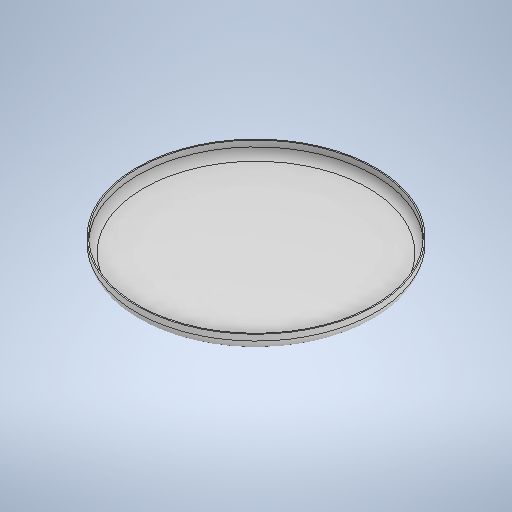
# Autodesk Inventor part: Сферическое дно D1000
Saved by Autodesk Inventor 2025 (Build 290162010, 162A)
## iProperties
Created: 2025-02-16
Part Number: Сферическое дно D1000
Material: Generic
Document SubType Name: Modeling
Designer: pokla
Density: 1 g/cm^3
Appearance: Default
Author: pokla
Autodesk Inventor part; units mm, degrees
ref_plane "YZ Plane" through (0, 0, 0) normal (1, 0, 0) x (0, 1, 0)
ref_plane "XZ Plane" through (0, 0, 0) normal (0, 1, 0) x (-1, 0, 0)
ref_plane "XY Plane" through (0, 0, 0) normal (0, 0, 1) x (1, 0, 0)
sketch "Sketch1" plane through (0, 0, 0) normal (0, 1, 0) x (-1, 0, 0)
  line L0 (606, 0) -> (606, -30)
  arc A0 (571.724, -77.4632) -> (606, -30) centre (556, -30) ccw
  arc A1 (0, -169.7009) -> (571.724, -77.4632) centre (0, 1648.2991) ccw
  line L1 (0, 191.6842) -> (0, -191.6842)
  arc A2 (0, -163.7009) -> (569.8371, -71.7676) centre (0, 1648.2991) ccw
  arc A3 (569.8371, -71.7676) -> (600, -30) centre (556, -30) ccw
  line L2 (600, -30) -> (600, 0)
  line L3 (600, 0) -> (606, 0)
  line L4 (0, -163.7009) -> (0, -169.7009)
  point P0 (0, 0)
  point P1 (0, 0)
  point P2 (0, -166.7009)
  point P3 (0, -163.7009)
  point P4 (0, -169.7009)
  dimension "d0" = 50
  dimension "d1" = 30
  dimension "d3" = 1818
  dimension "d4" = 606
  dimension "d6" = 6
  constraints: 10 end point, 8 point on circle, 4 centre point, 2 midpoint, 2 tangent, 2 vertical, 1 coincident, 1 horizontal, 1 horizontal alignment, 1 line through centre, 1 parallel, 1 vertical alignment, 2 other
  measures "d0" radius of A0
  measures "d1" distance of L0.start L0.end
  measures "d3" radius of A1
  measures "d4" distance of point (0, 0) L0.start
  measures "d6" radial gap between concentric circles of A1 A2
revolve "Revolution1" add sketch "Sketch1" angle 360 about axis through (0, 0, 191.6842) along (0, 0, -1)
body "Solid1"
